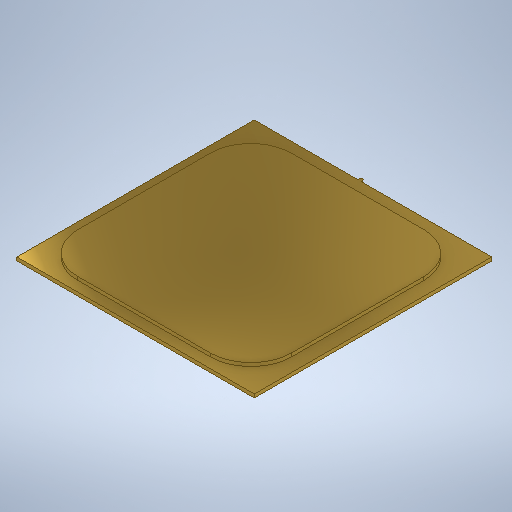
# Autodesk Inventor part: plate
Saved by Autodesk Inventor 2025 (Build 290162000, 162)
## iProperties
Created: 2025-09-08
Part Number: plate
Material: Gold
Document SubType Name: Modeling
Designer: jirne
Density: 19.3 g/cm^3
Appearance: Metal 1600F Hot
Author: jirne
Autodesk Inventor part; units mm, degrees
ref_plane "YZ Plane" through (0, 0, 0) normal (1, 0, 0) x (0, 1, 0)
ref_plane "XZ Plane" through (0, 0, 0) normal (0, 1, 0) x (-1, 0, 0)
ref_plane "XY Plane" through (0, 0, 0) normal (0, 0, 1) x (1, 0, 0)
sketch "Sketch1" plane through (0, 0, 0) normal (0, 0, 1) x (1, 0, 0)
  line L0 (0, 0) -> (17.78, 0)
  line L1 (17.78, 0) -> (17.78, 17.78)
  line L2 (17.78, 17.78) -> (0, 17.78)
  line L3 (0, 17.78) -> (0, 0)
  dimension "d0" = 17.78
  constraints: 8 end point, 2 parallel, 2 perpendicular, 1 horizontal
  measures "d0" distance of L2.end L0.start
extrude "Extrusion1" add sketch "Sketch1" along normal blind 0.254
sketch "Sketch2" plane through (0, 0, 0.254) normal (0, 0, 1) x (1, 0, 0)
  line L0 (0.762, 16.764) -> (16.764, 16.764)
  line L1 (16.764, 16.764) -> (16.764, 0.762)
  line L2 (16.764, 0.762) -> (0.762, 0.762)
  line L3 (0.762, 0.762) -> (0.762, 16.764)
  line L4 (0, 0) -> (17.78, 0) projected
  line L5 (0, 17.78) -> (0, 0) projected
  point P0 (0.762, 0.762)
  dimension "d3" = 16.002
  dimension "d4" = 0.762
  dimension "d5" = 0.762
  constraints: 8 end point, 2 parallel, 2 perpendicular, 1 horizontal
  measures "d3" distance of L2.end L0.start
  measures "d4" distance from line of L4 point (0.762, 0.762)
  measures "d5" distance from line of L5 point (0.762, 0.762)
extrude "Extrusion2" add sketch "Sketch2" along normal blind 0.254
fillet "Fillet1" radius 3.048 1 edges at (0.762, 0.762, 0.381)
fillet "Fillet2" radius 3.048 3 edges at (16.764, 0.762, 0.381) (16.764, 16.764, 0.381) (0.762, 16.764, 0.381)
sketch "Sketch3" plane through (0, 17.78, 0) normal (0, 1, 0) x (1, 0, 0)
  line L0 (17.78, 0) -> (0, 0) projected
  line L1 (0, -0.254) -> (17.78, -0.254) projected
  line L2 (7.747, 0) -> (8.001, 0)
  line L3 (8.001, 0) -> (8.001, -0.254)
  line L4 (8.001, -0.254) -> (7.747, -0.254)
  line L5 (7.747, -0.254) -> (7.747, 0)
  dimension "d10" = 7.747
  dimension "d11" = 0.254
  constraints: 8 end point, 2 parallel, 2 point on line, 1 horizontal, 1 perpendicular
  measures "d10" distance of L0.end L2.start
  measures "d11" distance between parallel lines of L5 L3
extrude "Extrusion3" add sketch "Sketch3" along normal blind 0.254
fillet "Fillet3" radius 0.127 2 edges at (8.001, 18.034, 0.127) (7.747, 18.034, 0.127)
body "Solid1"
